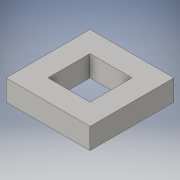
# Autodesk Inventor part: Peg Bottom
Saved by Autodesk Inventor 2016 (Build 200138000, 138)
## iProperties
Created: 2016-04-25
Part Number: Peg Bottom
Material: Generic
Document SubType Name: Modeling
Designer: rubenjm
Density: 1 g/cm^3
Appearance: Default
Author: rubenjm
Autodesk Inventor part; units mm, degrees
ref_plane "YZ Plane" through (0, 0, 0) normal (1, 0, 0) x (0, 1, 0)
ref_plane "XZ Plane" through (0, 0, 0) normal (0, 1, 0) x (-1, 0, 0)
ref_plane "XY Plane" through (0, 0, 0) normal (0, 0, 1) x (1, 0, 0)
sketch "Sketch1" plane through (0, 0, 0) normal (0, 1, 0) x (-1, 0, 0)
  line L0 (0, 0) -> (50.8, 0)
  line L1 (50.8, 0) -> (50.8, -50.8)
  line L2 (50.8, -50.8) -> (0, -50.8)
  line L3 (0, -50.8) -> (0, 0)
  line L4 (0, 0) -> (50.8, -50.8) construction
  line L5 (50.8, 0) -> (25.4, -25.4) construction
  line L6 (12.7, -12.7) -> (38.1, -12.7)
  line L7 (38.1, -12.7) -> (38.1, -38.1)
  line L8 (38.1, -38.1) -> (12.7, -38.1)
  line L9 (12.7, -38.1) -> (12.7, -12.7)
  line L10 (12.7, -12.7) -> (38.1, -38.1) construction
  line L11 (38.1, -12.7) -> (12.7, -38.1) construction
  dimension "d0" = 50.8
  dimension "d1" = 50.8
  dimension "d2" = 25.4
  dimension "d3" = 25.4
  constraints: 24 end point, 4 parallel, 3 midpoint, 2 horizontal, 2 perpendicular
  measures "d0" distance of L1.end L2.end
  measures "d1" distance of L0.end L1.end
  measures "d2" distance of L7.end L8.end
  measures "d3" distance of L6.end L7.end
extrude "Extrusion1" add sketch "Sketch1" along normal blind 12.7
body "Solid1"
